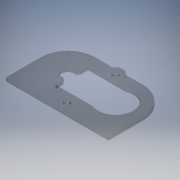
# Autodesk Inventor part: Dock top2 V2
Saved by Autodesk Inventor 2016 (Build 200138000, 138)
## iProperties
Created: 2017-03-31
Part Number: Dock top2 V2
Material: Acrylic
Document SubType Name: Modeling
Designer: Nanjar
Density: 1.188 g/cm^3
Appearance: Transparent - Clear
Author: Nanjar
Autodesk Inventor part; units mm, degrees
ref_plane "YZ Plane" through (0, 0, 0) normal (1, 0, 0) x (0, 1, 0)
ref_plane "XZ Plane" through (0, 0, 0) normal (0, 1, 0) x (-1, 0, 0)
ref_plane "XY Plane" through (0, 0, 0) normal (0, 0, 1) x (1, 0, 0)
sketch "Sketch1" plane through (0, 0, 0) normal (0, 1, 0) x (-1, 0, 0)
  arc A0 (-15, 0) -> (0, -15) centre (0, 0) ccw
  arc A1 (3.5986, 8.9) -> (3.5986, -8.9) centre (0, 0) ccw
  line L0 (24.0501, -8.9) -> (3.5986, -8.9)
  line L1 (0, -15) -> (9.6509, -15)
  arc A2 (9.6509, -15) -> (16.5791, -15) centre (13.115, -13) ccw
  circle A3 centre (13.115, 13.6) radius 1.5
  arc A4 (25.389, 3.3975) -> (24.0501, 4.7088) centre (20.7501, 0) ccw
  arc A5 (25.389, -3.3975) -> (25.389, 3.3975) centre (26.23, 0) ccw
  arc A6 (24.0501, -4.7088) -> (25.389, -3.3975) centre (20.7501, 0) ccw
  line L2 (24.0501, -4.7088) -> (24.0501, -8.9)
  line L3 (24.0501, -8.9) -> (3.5986, -8.9)
  arc A7 (3.5986, 8.9) -> (3.5986, -8.9) centre (0, 0) ccw
  line L4 (3.5986, 8.9) -> (24.0501, 8.9)
  line L5 (24.0501, 8.9) -> (24.0501, 4.7088)
  circle A8 centre (13.115, -13) radius 1.5
  line L6 (0, -15) -> (9.6509, -15)
  arc A9 (9.6509, -15) -> (16.5791, -15) centre (13.115, -13) ccw
  line L7 (16.5791, -15) -> (41.23, -15)
  line L8 (41.23, -15) -> (41.23, 18.9874)
  line L9 (41.23, 18.9874) -> (-15, 18.9874)
  line L10 (-15, 18.9874) -> (-15, 0)
  arc A10 (-15, 0) -> (0, -15) centre (0, 0) ccw
  line L11 (16.5791, -15) -> (41.23, -15)
  constraints: 24 end point, 18 point on circle, 11 centre point
extrude "Extrusion1" add sketch "Sketch1" along normal blind 2
fillet "Fillet1" radius 15 1 edges at (-41.23, 1, -15)
body "Solid1"
